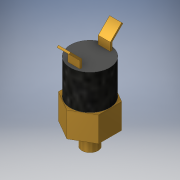
# Autodesk Inventor part: am-2006
Saved by Autodesk Inventor 2016 SP2 (Build 200236200, 236)
## iProperties
Created: 2017-03-28
Part Number: am-2006
Material: Brass
Document SubType Name: Modeling
Designer: smiku
Mass: 175.913 g
Surface Area: 62.4356 cm^2
Volume: 20.72 cm^3
Density: 8.49 g/cm^3
Appearance: Brass - Polished
Author: smiku
Autodesk Inventor part; units mm, degrees
ref_plane "YZ Plane" through (0, 0, 0) normal (1, 0, 0) x (0, 1, 0)
ref_plane "XZ Plane" through (0, 0, 0) normal (0, 1, 0) x (-1, 0, 0)
ref_plane "XY Plane" through (0, 0, 0) normal (0, 0, 1) x (1, 0, 0)
sketch "Sketch1" plane through (0, 0, 0) normal (0, 1, 0) x (-1, 0, 0)
  circle A0 centre (0, 0) radius 12.7 construction
  line L0 (12.7, -7.3323) -> (0, -14.6647)
  line L1 (0, -14.6647) -> (-12.7, -7.3323)
  line L2 (-12.7, -7.3323) -> (-12.7, 7.3323)
  line L3 (-12.7, 7.3323) -> (0, 14.6647)
  line L4 (0, 14.6647) -> (12.7, 7.3323)
  line L5 (12.7, 7.3323) -> (12.7, -7.3323)
  point P0 (12.7, 0)
  dimension "d0" = 25.4
  constraints: 12 end point, 2 coincident, 1 horizontal alignment, 1 midpoint, 1 vertical, 15 other
extrude "Extrusion1" add sketch "Sketch1" against normal blind 15.875
sketch "Sketch2" plane through (0, -15.875, 0) normal (0, -1, 0) x (1, 0, 0)
  circle A0 centre (0, 0) radius 1.5875
  circle A1 centre (0, 0) radius 5.08
  dimension "d3" = 3.175
  dimension "d4" = 10.16
  constraints: 2 centre point, 2 coincident
  measures "d3" diameter of A0
  measures "d4" diameter of A1
extrude "Extrusion2" add sketch "Sketch2" along normal blind 11.303
sketch "Sketch3" plane through (0, 0, 0) normal (0, 1, 0) x (1, 0, 0)
  circle A0 centre (0, 0) radius 12.446
  dimension "d7" = 24.892
  constraints: 1 centre point, 1 coincident
  measures "d7" diameter of A0
extrude "Extrusion3" add sketch "Sketch3" along normal blind 22.1234 separate body
sketch "Sketch4" plane through (0, 0, 0) normal (1, 0, 0) x (0, 1, 0)
  line L0 (22.1234, -12.446) -> (22.1234, 12.446) construction
  circle A0 centre (22.1234, 0) radius 9.0424 construction
  line L1 (22.1234, -9.0424) -> (27.2034, -9.0424)
  line L2 (22.1234, 9.0424) -> (27.2034, 9.0424)
  line L3 (27.2034, 9.0424) -> (34.3876, 16.2266)
  line L4 (27.2034, -9.0424) -> (34.3876, -16.2266)
  line L5 (27.2034, -9.0424) -> (37.3634, -9.0424) construction
  line L6 (33.5794, 17.0348) -> (26.73, 10.1854)
  line L7 (26.73, 10.1854) -> (22.1234, 10.1854)
  line L8 (33.5794, -17.0348) -> (26.73, -10.1854)
  line L9 (26.73, -10.1854) -> (22.1234, -10.1854)
  line L10 (22.1234, 10.1854) -> (22.1234, 9.0424)
  line L11 (22.1234, -9.0424) -> (22.1234, -10.1854)
  line L12 (34.3876, -16.2266) -> (33.5794, -17.0348)
  line L13 (34.3876, 16.2266) -> (33.5794, 17.0348)
  point P0 (0, 0)
  dimension "d10" = 18.0848
  dimension "d11" = 5.08
  dimension "d12" = 5.08
  dimension "d13" = 10.16
  dimension "d14" = 135
  dimension "d15" = 10.16
  dimension "d16" = 45
  dimension "d17" = 1.143
  dimension "d18" = 1.143
  constraints: 26 end point, 3 perpendicular, 2 collinear, 2 horizontal, 2 point on circle, 2 point on line, 2 tangent, 1 centre point, 1 equal length, 1 midpoint, 2 other
  measures "d10" diameter of A0
  measures "d11" distance of L1.start L1.end
  measures "d12" distance of L2.start L2.end
  measures "d13" distance of L2.end L3.end
  measures "d14" angle of L3 L2
  measures "d15" distance of L1.end L4.end
  measures "d16" angle of L4 L5
  measures "d17" distance between parallel lines of L3 L6
  measures "d18" distance between parallel lines of L4 L8
extrude "Extrusion4" add sketch "Sketch4" along normal mid plane 7.62 separate body
body "Solid1"
body "Solid2"
body "Solid3"
